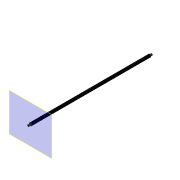
# Autodesk Inventor part: Part27
Saved by Autodesk Inventor 2016 (Build 200138000, 138)
## iProperties
Created: 2016-03-28
Part Number: Part27
Material: Aluminum 6061
Document SubType Name: Modeling
Designer: admin
Density: 2.71 g/cm^3
Appearance: Anodized - Black
Author: admin
Autodesk Inventor part; units mm, degrees
ref_plane "YZ Plane" through (0, 0, 0) normal (1, 0, 0) x (0, 1, 0)
ref_plane "XZ Plane" through (0, 0, 0) normal (0, 1, 0) x (-1, 0, 0)
ref_plane "XY Plane" through (0, 0, 0) normal (0, 0, 1) x (1, 0, 0)
ref_plane "Work Plane1" through (469.0633, -361.0645, -298.4444) normal (0, 1, 0) x (0, 0, 1)
sketch "Sketch2" plane through (469.0633, -361.0645, -298.4444) normal (0, 1, 0) x (0, 0, 1)
  circle A0 centre (0, 0) radius 3
  point P0 (298.4444, -469.0633)
  dimension "d6" = 6
  constraints: 1 centre point
  measures "d6" diameter of A0
extrude "Extrusion1" add sketch "Sketch2" along normal blind 251
sketch "Sketch5" plane through (469.0633, -110.0645, -298.4444) normal (0, 1, 0) x (1, 0, 0)
  circle A0 centre (0, 0) radius 3 projected
  circle A1 centre (0, 0) radius 1.5
  point P0 (-469.0633, -298.4444)
  dimension "d26" = 3
  constraints: 1 centre point, 1 coincident
  measures "d26" diameter of A1
extrude "Extrusion2" add sketch "Sketch5" along normal blind 4.7 contours A1
sketch "Sketch6" plane through (469.0633, -105.3645, -298.4444) normal (0, 1, 0) x (1, 0, 0)
  circle A0 centre (0, 0) radius 1.5 projected
  circle A1 centre (0, 0) radius 2
  point P0 (-469.0633, -298.4444)
  dimension "d29" = 4
  constraints: 1 centre point, 1 coincident
  measures "d29" diameter of A1
extrude "Extrusion3" add sketch "Sketch6" against normal blind 3.7
thread "Thread1" size "M4x0.7" class "6g" standard "ANSI Metric M Profile" full length
chamfer "Chamfer2" distance 0.3 angle 45 1 edges at (467.0633, -105.3645, -298.4444)
sketch "Sketch7" plane through (469.0633, -361.0645, -298.4444) normal (0, -1, 0) x (1, 0, 0)
  circle A0 centre (0, 0) radius 3 projected
  circle A1 centre (0, 0) radius 1.5
  point P0 (-469.0633, 298.4444)
  dimension "d37" = 3
  constraints: 1 centre point, 1 coincident
  measures "d37" diameter of A1
extrude "Extrusion4" add sketch "Sketch7" along normal blind 4.7 contours A1
sketch "Sketch8" plane through (469.0633, -365.7645, -298.4444) normal (0, -1, 0) x (1, 0, 0)
  circle A0 centre (0, 0) radius 1.5 projected
  circle A1 centre (0, 0) radius 2
  point P0 (-469.0633, 298.4444)
  dimension "d40" = 4
  constraints: 1 centre point, 1 coincident
  measures "d40" diameter of A1
extrude "Extrusion5" add sketch "Sketch8" against normal blind 3.7
thread "Thread2" size "M4x0.7" class "6g" standard "ANSI Metric M Profile" full length
chamfer "Chamfer3" distance 0.3 angle 45 1 edges at (467.0633, -365.7645, -298.4444)
body "Solid2"
